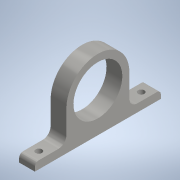
# Autodesk Inventor part: Soporte_Rodamiento
Saved by Autodesk Inventor 2022.1 (Build 261234000, 234)
## iProperties
Part Number: Soporte_Rodamiento
Material: Genérico
Document SubType Name: Modelado
Designer: seb_0
Appearance: Acero
Author: seb_0
Autodesk Inventor part; units mm, degrees
ref_plane "Plano YZ" through (0, 0, 0) normal (1, 0, 0) x (0, 1, 0)
ref_plane "Plano XZ" through (0, 0, 0) normal (0, 1, 0) x (-1, 0, 0)
ref_plane "Plano XY" through (0, 0, 0) normal (0, 0, 1) x (1, 0, 0)
sketch "Boceto3" plane through (0, 0, 0) normal (1, 0, 0) x (0, 1, 0)
  circle A0 centre (0, 0) radius 31
  circle A1 centre (0, 0) radius 40
  line L0 (-49.5, 80) -> (-49.5, -80)
  line L1 (-49.5, 80) -> (-44.5, 80)
  line L2 (-39.5, 75) -> (-39.5, 50)
  line L3 (-29.5, 40) -> (0, 40)
  line L4 (0, -40) -> (-29.5, -40)
  line L5 (-39.5, -50) -> (-39.5, -75)
  line L6 (-44.5, -80) -> (-49.5, -80)
  arc A2 (-39.5, 75) -> (-44.5, 80) centre (-44.5, 75) ccw
  arc A3 (-44.5, -80) -> (-39.5, -75) centre (-44.5, -75) ccw
  arc A4 (-39.5, 50) -> (-29.5, 40) centre (-29.5, 50) ccw
  arc A5 (-29.5, -40) -> (-39.5, -50) centre (-29.5, -50) ccw
  point P0 (-39.5, 80)
  point P1 (-39.5, -40)
  point P2 (-39.5, -80)
  dimension "d26" = 62
  dimension "d27" = 80
  dimension "d28" = 160
  dimension "d29" = 49.5
  dimension "d30" = 10
  dimension "d31" = 5
  dimension "d32" = 5
  dimension "d33" = 10
  constraints: 14 end point, 10 point on circle, 10 tangent, 8 point on line, 6 centre point, 2 coincident, 2 equal length, 2 perpendicular, 1 equal radius, 1 horizontal, 1 parallel, 1 vertical
  measures "d26" diameter of A0
  measures "d27" diameter of A1
  measures "d28" distance of L0.start L0.end
  measures "d29" distance from line of L0 point (0, 0)
  measures "d30" distance of L0.start point (-39.5, 80)
  measures "d31" radius of A2
  measures "d32" radius of A3
  measures "d33" radius of A4
extrude "Extrusión3" add sketch "Boceto3" along normal blind 20
sketch "Boceto4" plane through (0, -39.5, 75) normal (0, 1, 0) x (1, 0, 0)
  circle A0 centre (10, 10) radius 4
  circle A1 centre (10, 140) radius 4
  line L0 (20, 150) -> (20, 125) projected
  line L1 (0, 155) -> (20, 155) projected
  line L2 (20, 25) -> (20, 0) projected
  line L3 (0, -5) -> (20, -5) projected
  point P0 (0, 75)
  dimension "d36" = 8
  dimension "d37" = 8
  dimension "d38" = 10
  dimension "d39" = 15
  dimension "d40" = 10
  dimension "d41" = 15
  constraints: 2 centre point
  measures "d36" diameter of A0
  measures "d37" diameter of A1
  measures "d38" distance from line of A1.centre L0
  measures "d39" distance from line of L1 A1.centre
  measures "d40" distance from line of L2 A0.centre
  measures "d41" distance from line of A0.centre L3
extrude "Extrusión4" cut sketch "Boceto4" against normal through all
